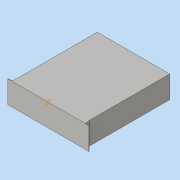
# Autodesk Inventor part: monitorControl
Saved by Autodesk Inventor 2016 (Build 200138000, 138)
## iProperties
Created: 2016-08-08
Part Number: monitorControl
Material: Generic
Document SubType Name: Modeling
Designer: Zuhra Abdurashidova
Density: 1 g/cm^3
Appearance: Default
Sheet Metal Rule: Default
Author: Zuhra Abdurashidova
Autodesk Inventor part; units mm, degrees
ref_plane "YZ Plane" through (0, 0, 0) normal (1, 0, 0) x (0, 1, 0)
ref_plane "XZ Plane" through (0, 0, 0) normal (0, 1, 0) x (-1, 0, 0)
ref_plane "XY Plane" through (0, 0, 0) normal (0, 0, 1) x (1, 0, 0)
sketch "Sketch2" plane through (0, 0, 0) normal (0, 1, 0) x (-1, 0, 0)
  line L0 (215.9, 254) -> (-215.9, 254)
  line L1 (-215.9, 254) -> (-215.9, -254)
  line L2 (-215.9, -254) -> (215.9, -254)
  line L3 (215.9, -254) -> (215.9, 254)
  line L4 (215.9, 254) -> (-215.9, -254) construction
  line L5 (-215.9, 254) -> (215.9, -254) construction
  point P0 (0, 0)
  point P1 (0, -254)
  dimension "d6" = 431.8
  dimension "d7" = 508
  constraints: 12 end point, 3 midpoint, 2 parallel, 1 horizontal, 1 perpendicular
  measures "d6" distance of L1.end L2.end
  measures "d7" distance of L0.end L1.end
extrude "Extrusion3" add sketch "Sketch2" along normal blind 133.35
ref_plane "Work Plane3" through (0, 133.35, 254) normal (1, 0, 0) x (0, 1, 0)
sketch "Sketch4" plane through (0, 133.35, 0) normal (0, 1, 0) x (1, 0, 0)
  line L0 (-215.9, -254) -> (215.9, -254) projected
  line L1 (215.9, -228.6) -> (215.9, -254)
  line L2 (215.9, -254) -> (241.3, -254)
  line L3 (241.3, -251.3584) -> (218.5416, -251.3584)
  line L4 (218.5416, -251.3584) -> (218.5416, -228.6)
  line L5 (215.9, -228.6) -> (218.5416, -228.6)
  line L6 (215.9, -254) -> (215.9, 254) projected
  line L7 (241.3, -254) -> (241.3, -251.3584)
  point P0 (0, 0)
  dimension "d13" = 25.4
  dimension "d14" = 25.4
  dimension "d15" = 2.6416
  constraints: 12 end point, 4 perpendicular, 1 vertical, 1 other
  measures "d13" distance of L0.end L2.end
  measures "d14" distance of L1.start L0.end
  measures "d15" distance between parallel lines of L3 L2
extrude "Extrusion5" add sketch "Sketch4" against normal blind 133.35
mirror "Mirror1" about plane through (0, 133.35, 254) normal (1, 0, 0) of "Extrusion5"
equation "\"BendRadius\" = Thickness"
equation "\"BendReliefWidth\" = Thickness"
equation "\"BendReliefDepth\" = 0.5 * Thickness"
equation "\"CornerReliefSize\" = 4 * Thickness"
equation "\"MinimumRemnant\" = 2 * Thickness"
equation "\"TransitionRadius\" = BendRadius"
equation "\"JacobiRadiusSize\" = Thickness"
equation "\"GapSize\" = Thickness"
equation "\"Thickness\" = 3.048"
body "Solid3"
